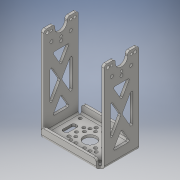
# Autodesk Inventor part: PahaAtas
Saved by Autodesk Inventor 2016 (Build 200138000, 138)
## iProperties
Created: 2017-02-10
Part Number: PahaAtas
Material: Generic
Document SubType Name: Modeling
Designer: Ghana
Density: 1 g/cm^3
Appearance: Default
Author: Ghana
Autodesk Inventor part; units mm, degrees
note: some values were not read from the file. Chosen so that the rebuilt part matches the saved one: bend side of "Bend Part10"; bend side of "Bend Part11".
ref_plane "YZ Plane" through (0, 0, 0) normal (1, 0, 0) x (0, 1, 0)
ref_plane "XZ Plane" through (0, 0, 0) normal (0, 1, 0) x (-1, 0, 0)
ref_plane "XY Plane" through (0, 0, 0) normal (0, 0, 1) x (1, 0, 0)
sketch "Sketch12" plane through (0, 0, 0) normal (0, 1, 0) x (-1, 0, 0)
  line L0 (0, 0) -> (44.454, 0)
  line L1 (44.454, 0) -> (44.454, -28)
  line L2 (44.454, -28) -> (0, -28)
  line L3 (0, -28) -> (0, 0)
  line L4 (44.454, 0) -> (46.454, 0)
  line L5 (46.454, 0) -> (46.454, -28)
  line L6 (46.454, -28) -> (44.454, -28)
  line L7 (44.454, -28) -> (44.454, 0)
  line L8 (0, 0) -> (-2, 0)
  line L9 (-2, 0) -> (-2, -28)
  line L10 (-2, -28) -> (0, -28)
  line L11 (0, -28) -> (0, 0)
  line L12 (46.454, 0) -> (115.181, 0)
  line L13 (117.181, -2) -> (117.181, -7)
  line L14 (115.181, -28) -> (46.454, -28)
  line L15 (46.454, -28) -> (46.454, 0)
  line L16 (-2, -28) -> (-70.727, -28)
  line L17 (-2, 0) -> (-2, -28)
  circle A0 centre (22.227, -14) radius 5.2
  circle A1 centre (22.227, -3) radius 1.25
  circle A2 centre (30.0052, -6.2218) radius 1.25
  circle A3 centre (33.227, -14) radius 1.25
  circle A4 centre (30.0052, -21.7782) radius 1.25
  circle A5 centre (22.227, -25) radius 1.25
  circle A6 centre (14.4488, -21.7782) radius 1.25
  circle A7 centre (11.227, -14) radius 1.25
  circle A8 centre (14.4488, -6.2218) radius 1.25
  circle A9 centre (25.727, -6) radius 1.35
  circle A10 centre (14.227, -10.5) radius 1.35
  circle A11 centre (18.727, -22) radius 1.35
  circle A12 centre (30.227, -17.5) radius 1.35
  circle A13 centre (18.727, -6) radius 1.25
  circle A14 centre (14.227, -17.5) radius 1.25
  circle A15 centre (25.727, -22) radius 1.25
  circle A16 centre (30.227, -10.5) radius 1.25
  circle A17 centre (33.227, -8) radius 1.35
  circle A18 centre (16.227, -3) radius 1.35
  circle A19 centre (11.227, -20) radius 1.35
  circle A20 centre (28.227, -25) radius 1.35
  circle A21 centre (11.227, -8) radius 1.25
  circle A22 centre (16.227, -25) radius 1.25
  circle A23 centre (33.227, -20) radius 1.25
  circle A24 centre (28.227, -3) radius 1.25
  circle A25 centre (3.227, -25) radius 1.25
  circle A26 centre (41.227, -25) radius 1.25
  circle A27 centre (3.227, -3) radius 1.25
  circle A28 centre (41.227, -3) radius 1.25
  line L18 (37.727, -9) -> (39.227, -9)
  arc A29 (40.727, -10.5) -> (39.227, -9) centre (39.227, -10.5) ccw
  line L19 (40.727, -10.5) -> (40.727, -17.5)
  arc A30 (39.227, -19) -> (40.727, -17.5) centre (39.227, -17.5) ccw
  line L20 (39.227, -19) -> (37.727, -19)
  arc A31 (36.227, -17.5) -> (37.727, -19) centre (37.727, -17.5) ccw
  line L21 (36.227, -17.5) -> (36.227, -10.5)
  arc A32 (37.727, -9) -> (36.227, -10.5) centre (37.727, -10.5) ccw
  line L22 (8.227, -10.5) -> (8.227, -17.5)
  arc A33 (6.727, -19) -> (8.227, -17.5) centre (6.727, -17.5) ccw
  line L23 (6.727, -19) -> (5.227, -19)
  arc A34 (3.727, -17.5) -> (5.227, -19) centre (5.227, -17.5) ccw
  line L24 (3.727, -17.5) -> (3.727, -10.5)
  arc A35 (5.227, -9) -> (3.727, -10.5) centre (5.227, -10.5) ccw
  line L25 (5.227, -9) -> (6.727, -9)
  arc A36 (8.227, -10.5) -> (6.727, -9) centre (6.727, -10.5) ccw
  line L26 (44.454, -28) -> (0, -28)
  line L27 (0, -28) -> (0, -30)
  line L28 (0, -30) -> (44.454, -30)
  line L29 (44.454, -30) -> (44.454, -28)
  line L30 (44.454, 0) -> (0, 0)
  line L31 (0, 0) -> (0, 2)
  line L32 (0, 2) -> (44.454, 2)
  line L33 (44.454, 2) -> (44.454, 0)
  line L34 (44.454, -30) -> (0, -30)
  line L35 (0, -30) -> (0, -33)
  line L36 (2, -35) -> (42.454, -35)
  line L37 (44.454, -33) -> (44.454, -30)
  line L38 (44.454, 2) -> (0, 2)
  line L39 (0, 2) -> (0, 5)
  line L40 (2, 7) -> (42.454, 7)
  line L41 (44.454, 5) -> (44.454, 2)
  arc A37 (42.454, -35) -> (44.454, -33) centre (42.454, -33) ccw
  arc A38 (0, -33) -> (2, -35) centre (2, -33) ccw
  arc A39 (44.454, 5) -> (42.454, 7) centre (42.454, 5) ccw
  arc A40 (2, 7) -> (0, 5) centre (2, 5) ccw
  line L42 (114.181, -19) -> (115.181, -19)
  line L43 (114.181, -9) -> (115.181, -9)
  arc A41 (114.181, -9) -> (114.181, -19) centre (114.181, -14) ccw
  line L44 (117.181, -21) -> (117.181, -26)
  circle A42 centre (114.181, -25) radius 1.25
  circle A43 centre (114.181, -22) radius 1
  circle A44 centre (106.4028, -21.7782) radius 1.25
  circle A45 centre (103.181, -14) radius 1.25
  circle A46 centre (106.4028, -6.2218) radius 1.25
  circle A47 centre (114.181, -3) radius 1.25
  circle A48 centre (106.181, -14) radius 1
  circle A49 centre (114.181, -6) radius 1
  line L45 (53.454, -8.7321) -> (53.454, -19.2679)
  line L46 (54.954, -20.134) -> (64.0784, -14.866)
  line L47 (64.0784, -13.134) -> (54.954, -7.866)
  line L48 (98.181, -19.2679) -> (98.181, -8.7321)
  line L49 (96.681, -20.134) -> (87.5566, -14.866)
  line L50 (87.5566, -13.134) -> (96.681, -7.866)
  line L51 (86.9131, -23) -> (64.7219, -23)
  line L52 (64.2219, -21.134) -> (74.8175, -15.0166)
  line L53 (76.8175, -15.0166) -> (87.4131, -21.134)
  line L54 (76.8175, -12.9834) -> (87.4131, -6.866)
  line L55 (86.9131, -5) -> (64.7219, -5)
  line L56 (64.2219, -6.866) -> (74.8175, -12.9834)
  arc A50 (74.8175, -12.9834) -> (76.8175, -12.9834) centre (75.8175, -11.2513) ccw
  arc A51 (76.8175, -15.0166) -> (74.8175, -15.0166) centre (75.8175, -16.7487) ccw
  arc A52 (96.681, -20.134) -> (98.181, -19.2679) centre (97.181, -19.2679) ccw
  arc A53 (98.181, -8.7321) -> (96.681, -7.866) centre (97.181, -8.7321) ccw
  arc A54 (87.5566, -13.134) -> (87.5566, -14.866) centre (88.0566, -14) ccw
  arc A55 (86.9131, -23) -> (87.4131, -21.134) centre (86.9131, -22) ccw
  arc A56 (64.2219, -21.134) -> (64.7219, -23) centre (64.7219, -22) ccw
  arc A57 (87.4131, -6.866) -> (86.9131, -5) centre (86.9131, -6) ccw
  arc A58 (64.7219, -5) -> (64.2219, -6.866) centre (64.7219, -6) ccw
  arc A59 (64.0784, -14.866) -> (64.0784, -13.134) centre (63.5784, -14) ccw
  arc A60 (53.454, -19.2679) -> (54.954, -20.134) centre (54.454, -19.2679) ccw
  arc A61 (54.954, -7.866) -> (53.454, -8.7321) centre (54.454, -8.7321) ccw
  line L57 (-9, -8.7321) -> (-9, -19.2679)
  line L58 (-10.5, -20.134) -> (-19.6244, -14.866)
  line L59 (-19.6244, -13.134) -> (-10.5, -7.866)
  line L60 (-53.727, -19.2679) -> (-53.727, -8.7321)
  line L61 (-52.227, -20.134) -> (-43.1026, -14.866)
  line L62 (-43.1026, -13.134) -> (-52.227, -7.866)
  line L63 (-42.4591, -23) -> (-20.2679, -23)
  line L64 (-19.7679, -21.134) -> (-30.3635, -15.0166)
  line L65 (-32.3635, -15.0166) -> (-42.9591, -21.134)
  line L66 (-32.3635, -12.9834) -> (-42.9591, -6.866)
  line L67 (-42.4591, -5) -> (-20.2679, -5)
  line L68 (-19.7679, -6.866) -> (-30.3635, -12.9834)
  arc A62 (-32.3635, -12.9834) -> (-30.3635, -12.9834) centre (-31.3635, -11.2513) ccw
  arc A63 (-30.3635, -15.0166) -> (-32.3635, -15.0166) centre (-31.3635, -16.7487) ccw
  arc A64 (-53.727, -19.2679) -> (-52.227, -20.134) centre (-52.727, -19.2679) ccw
  arc A65 (-52.227, -7.866) -> (-53.727, -8.7321) centre (-52.727, -8.7321) ccw
  arc A66 (-43.1026, -14.866) -> (-43.1026, -13.134) centre (-43.6026, -14) ccw
  arc A67 (-42.9591, -21.134) -> (-42.4591, -23) centre (-42.4591, -22) ccw
  arc A68 (-20.2679, -23) -> (-19.7679, -21.134) centre (-20.2679, -22) ccw
  arc A69 (-42.4591, -5) -> (-42.9591, -6.866) centre (-42.4591, -6) ccw
  arc A70 (-19.7679, -6.866) -> (-20.2679, -5) centre (-20.2679, -6) ccw
  arc A71 (-19.6244, -13.134) -> (-19.6244, -14.866) centre (-19.1244, -14) ccw
  arc A72 (-10.5, -20.134) -> (-9, -19.2679) centre (-10, -19.2679) ccw
  arc A73 (-9, -8.7321) -> (-10.5, -7.866) centre (-10, -8.7321) ccw
  arc A74 (115.181, -28) -> (117.181, -26) centre (115.181, -26) ccw
  arc A75 (117.181, -21) -> (115.181, -19) centre (115.181, -21) ccw
  arc A76 (115.181, -9) -> (117.181, -7) centre (115.181, -7) ccw
  arc A77 (117.181, -2) -> (115.181, 0) centre (115.181, -2) ccw
  line L69 (-72.727, -2) -> (-72.727, -7)
  line L70 (-69.727, -19) -> (-70.727, -19)
  line L71 (-69.727, -9) -> (-70.727, -9)
  arc A78 (-69.727, -19) -> (-69.727, -9) centre (-69.727, -14) ccw
  line L72 (-72.727, -21) -> (-72.727, -26)
  circle A79 centre (-69.727, -25) radius 1.25
  circle A80 centre (-69.727, -22) radius 1
  circle A81 centre (-61.9488, -21.7782) radius 1.25
  circle A82 centre (-58.727, -14) radius 1.25
  circle A83 centre (-61.9488, -6.2218) radius 1.25
  circle A84 centre (-69.727, -3) radius 1.25
  circle A85 centre (-61.727, -14) radius 1
  circle A86 centre (-69.727, -6) radius 1
  arc A87 (-72.727, -26) -> (-70.727, -28) centre (-70.727, -26) ccw
  arc A88 (-70.727, -19) -> (-72.727, -21) centre (-70.727, -21) ccw
  arc A89 (-72.727, -7) -> (-70.727, -9) centre (-70.727, -7) ccw
  arc A90 (-70.727, 0) -> (-72.727, -2) centre (-70.727, -2) ccw
  line L73 (-70.727, 0) -> (-2, 0)
  point P0 (117.181, -28)
  point P1 (117.181, 0)
  point P2 (22.227, -14)
  point P3 (0, -35)
  point P4 (0, 7)
  dimension "d88" = 2
  dimension "d89" = 2
  dimension "d91" = 70.727
  dimension "d92" = 28
  dimension "d97" = 44.454
  dimension "d98" = 2
  dimension "d99" = 44.454
  dimension "d100" = 2
  dimension "d101" = 5
  dimension "d102" = 5
  dimension "d103" = 2
  dimension "d114" = 180
  dimension "d118" = 180
  dimension "d132" = 2
  constraints: 148 end point, 92 point on circle, 91 centre point, 40 tangent, 18 parallel, 16 equal radius, 9 horizontal, 9 perpendicular, 9 point on line, 1 vertical, 14 other
  measures "d88" distance of L5.end L6.end
  measures "d89" distance of L10.end L9.end
  measures "d91" distance of point (117.181, -28) L14.end
  measures "d92" distance of point (117.181, 0) point (117.181, -28)
  measures "d97" distance of L28.end L27.end
  measures "d98" distance of L27.end L26.end
  measures "d99" distance of L31.end L32.end
  measures "d100" distance of L30.end L31.end
  measures "d101" distance of point (0, -35) L34.end
  measures "d102" distance of L38.end point (0, 7)
  measures "d103" radius of A37
  measures "d132" radius of A74
extrude "Extrusion6" add sketch "Sketch12" along normal blind 2
sketch "Sketch17" plane through (0, 2, 0) normal (0, 1, 0) x (1, 0, 0)
  arc A0 (30.3635, 15.0166) -> (32.3635, 15.0166) centre (31.3635, 16.7487) ccw projected
  line L0 (30.3635, 15.0166) -> (19.7679, 21.134) projected
  arc A1 (20.2679, 23) -> (19.7679, 21.134) centre (20.2679, 22) ccw projected
  line L1 (20.2679, 23) -> (42.4591, 23) projected
  arc A2 (42.9591, 21.134) -> (42.4591, 23) centre (42.4591, 22) ccw projected
  line L2 (42.9591, 21.134) -> (32.3635, 15.0166) projected
  arc A3 (19.7679, 6.866) -> (20.2679, 5) centre (20.2679, 6) ccw projected
  line L3 (19.7679, 6.866) -> (30.3635, 12.9834) projected
  arc A4 (32.3635, 12.9834) -> (30.3635, 12.9834) centre (31.3635, 11.2513) ccw projected
  line L4 (32.3635, 12.9834) -> (42.9591, 6.866) projected
  arc A5 (42.4591, 5) -> (42.9591, 6.866) centre (42.4591, 6) ccw projected
  line L5 (42.4591, 5) -> (20.2679, 5) projected
  arc A6 (52.227, 7.866) -> (53.727, 8.7321) centre (52.727, 8.7321) ccw projected
  line L6 (52.227, 7.866) -> (43.1026, 13.134) projected
  arc A7 (43.1026, 14.866) -> (43.1026, 13.134) centre (43.6026, 14) ccw projected
  line L7 (43.1026, 14.866) -> (52.227, 20.134) projected
  arc A8 (53.727, 19.2679) -> (52.227, 20.134) centre (52.727, 19.2679) ccw projected
  line L8 (53.727, 19.2679) -> (53.727, 8.7321) projected
  arc A9 (10.5, 20.134) -> (9, 19.2679) centre (10, 19.2679) ccw projected
  line L9 (10.5, 20.134) -> (19.6244, 14.866) projected
  arc A10 (19.6244, 13.134) -> (19.6244, 14.866) centre (19.1244, 14) ccw projected
  line L10 (19.6244, 13.134) -> (10.5, 7.866) projected
  arc A11 (9, 8.7321) -> (10.5, 7.866) centre (10, 8.7321) ccw projected
  line L11 (9, 8.7321) -> (9, 19.2679) projected
  circle A12 centre (61.9488, 6.2218) radius 1.25 projected
  circle A13 centre (69.727, 3) radius 1.25 projected
  circle A14 centre (58.727, 14) radius 1.25 projected
  circle A15 centre (69.727, 25) radius 1.25 projected
  circle A16 centre (61.9488, 21.7782) radius 1.25 projected
  circle A17 centre (69.727, 6) radius 1 projected
  circle A18 centre (61.727, 14) radius 1 projected
  circle A19 centre (69.727, 22) radius 1 projected
  arc A20 (-76.8175, 15.0166) -> (-74.8175, 15.0166) centre (-75.8175, 16.7487) ccw projected
  line L12 (-76.8175, 15.0166) -> (-87.4131, 21.134) projected
  arc A21 (-86.9131, 23) -> (-87.4131, 21.134) centre (-86.9131, 22) ccw projected
  line L13 (-86.9131, 23) -> (-64.7219, 23) projected
  arc A22 (-64.2219, 21.134) -> (-64.7219, 23) centre (-64.7219, 22) ccw projected
  line L14 (-64.2219, 21.134) -> (-74.8175, 15.0166) projected
  arc A23 (-64.7219, 5) -> (-64.2219, 6.866) centre (-64.7219, 6) ccw projected
  line L15 (-64.7219, 5) -> (-86.9131, 5) projected
  arc A24 (-87.4131, 6.866) -> (-86.9131, 5) centre (-86.9131, 6) ccw projected
  line L16 (-87.4131, 6.866) -> (-76.8175, 12.9834) projected
  arc A25 (-74.8175, 12.9834) -> (-76.8175, 12.9834) centre (-75.8175, 11.2513) ccw projected
  line L17 (-74.8175, 12.9834) -> (-64.2219, 6.866) projected
  arc A26 (-53.454, 19.2679) -> (-54.954, 20.134) centre (-54.454, 19.2679) ccw projected
  line L18 (-53.454, 19.2679) -> (-53.454, 8.7321) projected
  arc A27 (-54.954, 7.866) -> (-53.454, 8.7321) centre (-54.454, 8.7321) ccw projected
  line L19 (-54.954, 7.866) -> (-64.0784, 13.134) projected
  arc A28 (-64.0784, 14.866) -> (-64.0784, 13.134) centre (-63.5784, 14) ccw projected
  line L20 (-64.0784, 14.866) -> (-54.954, 20.134) projected
  arc A29 (-96.681, 20.134) -> (-98.181, 19.2679) centre (-97.181, 19.2679) ccw projected
  line L21 (-96.681, 20.134) -> (-87.5566, 14.866) projected
  arc A30 (-87.5566, 13.134) -> (-87.5566, 14.866) centre (-88.0566, 14) ccw projected
  line L22 (-87.5566, 13.134) -> (-96.681, 7.866) projected
  arc A31 (-98.181, 8.7321) -> (-96.681, 7.866) centre (-97.181, 8.7321) ccw projected
  line L23 (-98.181, 8.7321) -> (-98.181, 19.2679) projected
  circle A32 centre (-114.181, 3) radius 1.25 projected
  circle A33 centre (-106.4028, 6.2218) radius 1.25 projected
  circle A34 centre (-103.181, 14) radius 1.25 projected
  circle A35 centre (-106.4028, 21.7782) radius 1.25 projected
  circle A36 centre (-114.181, 25) radius 1.25 projected
  circle A37 centre (-114.181, 6) radius 1 projected
  circle A38 centre (-106.181, 14) radius 1 projected
  circle A39 centre (-114.181, 22) radius 1 projected
  circle A40 centre (-22.227, 14) radius 5.2 projected
  arc A41 (-6.727, 19) -> (-8.227, 17.5) centre (-6.727, 17.5) ccw projected
  line L24 (-6.727, 19) -> (-5.227, 19) projected
  arc A42 (-3.727, 17.5) -> (-5.227, 19) centre (-5.227, 17.5) ccw projected
  line L25 (-3.727, 17.5) -> (-3.727, 10.5) projected
  arc A43 (-5.227, 9) -> (-3.727, 10.5) centre (-5.227, 10.5) ccw projected
  line L26 (-5.227, 9) -> (-6.727, 9) projected
  arc A44 (-8.227, 10.5) -> (-6.727, 9) centre (-6.727, 10.5) ccw projected
  line L27 (-8.227, 10.5) -> (-8.227, 17.5) projected
  arc A45 (-40.727, 10.5) -> (-39.227, 9) centre (-39.227, 10.5) ccw projected
  line L28 (-40.727, 10.5) -> (-40.727, 17.5) projected
  arc A46 (-39.227, 19) -> (-40.727, 17.5) centre (-39.227, 17.5) ccw projected
  line L29 (-39.227, 19) -> (-37.727, 19) projected
  arc A47 (-36.227, 17.5) -> (-37.727, 19) centre (-37.727, 17.5) ccw projected
  line L30 (-36.227, 17.5) -> (-36.227, 10.5) projected
  arc A48 (-37.727, 9) -> (-36.227, 10.5) centre (-37.727, 10.5) ccw projected
  line L31 (-37.727, 9) -> (-39.227, 9) projected
  circle A49 centre (-28.227, 25) radius 1.35 projected
  circle A50 centre (-11.227, 20) radius 1.35 projected
  circle A51 centre (-16.227, 3) radius 1.35 projected
  circle A52 centre (-33.227, 8) radius 1.35 projected
  circle A53 centre (-30.227, 17.5) radius 1.35 projected
  circle A54 centre (-18.727, 22) radius 1.35 projected
  circle A55 centre (-14.227, 10.5) radius 1.35 projected
  circle A56 centre (-25.727, 6) radius 1.35 projected
  circle A57 centre (-41.227, 3) radius 1.25 projected
  circle A58 centre (-3.227, 3) radius 1.25 projected
  circle A59 centre (-41.227, 25) radius 1.25 projected
  circle A60 centre (-3.227, 25) radius 1.25 projected
  circle A61 centre (-28.227, 3) radius 1.25 projected
  circle A62 centre (-33.227, 20) radius 1.25 projected
  circle A63 centre (-16.227, 25) radius 1.25 projected
  circle A64 centre (-11.227, 8) radius 1.25 projected
  circle A65 centre (-30.227, 10.5) radius 1.25 projected
  circle A66 centre (-25.727, 22) radius 1.25 projected
  circle A67 centre (-14.227, 17.5) radius 1.25 projected
  circle A68 centre (-18.727, 6) radius 1.25 projected
  circle A69 centre (-14.4488, 6.2218) radius 1.25 projected
  circle A70 centre (-11.227, 14) radius 1.25 projected
  circle A71 centre (-14.4488, 21.7782) radius 1.25 projected
  circle A72 centre (-22.227, 25) radius 1.25 projected
  circle A73 centre (-30.0052, 21.7782) radius 1.25 projected
  circle A74 centre (-33.227, 14) radius 1.25 projected
  circle A75 centre (-30.0052, 6.2218) radius 1.25 projected
  circle A76 centre (-22.227, 3) radius 1.25 projected
  line L32 (-44.454, 28) -> (-115.181, 28) projected
  arc A77 (-115.181, 28) -> (-117.181, 26) centre (-115.181, 26) ccw projected
  line L33 (-117.181, 26) -> (-117.181, 21) projected
  arc A78 (-117.181, 21) -> (-115.181, 19) centre (-115.181, 21) ccw projected
  line L34 (-115.181, 19) -> (-114.181, 19) projected
  arc A79 (-114.181, 9) -> (-114.181, 19) centre (-114.181, 14) ccw projected
  line L35 (-114.181, 9) -> (-115.181, 9) projected
  arc A80 (-115.181, 9) -> (-117.181, 7) centre (-115.181, 7) ccw projected
  line L36 (-117.181, 7) -> (-117.181, 2) projected
  arc A81 (-117.181, 2) -> (-115.181, 0) centre (-115.181, 2) ccw projected
  line L37 (-115.181, 0) -> (-44.454, 0) projected
  line L38 (-44.454, 0) -> (-44.454, -5) projected
  arc A82 (-44.454, -5) -> (-42.454, -7) centre (-42.454, -5) ccw projected
  line L39 (-42.454, -7) -> (-2, -7) projected
  arc A83 (-2, -7) -> (0, -5) centre (-2, -5) ccw projected
  line L40 (0, -5) -> (0, 0) projected
  line L41 (0, 0) -> (70.727, 0) projected
  arc A84 (70.727, 0) -> (72.727, 2) centre (70.727, 2) ccw projected
  line L42 (72.727, 2) -> (72.727, 7) projected
  arc A85 (72.727, 7) -> (70.727, 9) centre (70.727, 7) ccw projected
  line L43 (70.727, 9) -> (69.727, 9) projected
  arc A86 (69.727, 19) -> (69.727, 9) centre (69.727, 14) ccw projected
  line L44 (69.727, 19) -> (70.727, 19) projected
  arc A87 (70.727, 19) -> (72.727, 21) centre (70.727, 21) ccw projected
  line L45 (72.727, 21) -> (72.727, 26) projected
  arc A88 (72.727, 26) -> (70.727, 28) centre (70.727, 26) ccw projected
  line L46 (70.727, 28) -> (0, 28) projected
  line L47 (0, 28) -> (0, 33) projected
  arc A89 (0, 33) -> (-2, 35) centre (-2, 33) ccw projected
  line L48 (-2, 35) -> (-42.454, 35) projected
  arc A90 (-42.454, 35) -> (-44.454, 33) centre (-42.454, 33) ccw projected
  line L49 (-44.454, 33) -> (-44.454, 28) projected
  line L50 (-44.454, 28) -> (-44.454, 0)
  constraints: 2 end point, 1 vertical
bend part "Bend Part9" radius 1.2732 angle 90 line through (-44.454, 2, -28) along (0, 0, 1) centre toward (0, 1, 0) moving side (-1, 0, 0) both sides no
sketch "Sketch18" plane through (0, 2, 0) normal (0, 1, 0) x (1, 0, 0)
  line L0 (-44.454, 0) -> (-44.454, 28) projected
  line L1 (-44.454, 0) -> (-44.454, -5) projected
  arc A0 (-44.454, -5) -> (-42.454, -7) centre (-42.454, -5) ccw projected
  line L2 (-42.454, -7) -> (-2, -7) projected
  arc A1 (-2, -7) -> (0, -5) centre (-2, -5) ccw projected
  line L3 (0, -5) -> (0, 0) projected
  line L4 (0, 0) -> (70.727, 0) projected
  arc A2 (70.727, 0) -> (72.727, 2) centre (70.727, 2) ccw projected
  line L5 (72.727, 2) -> (72.727, 7) projected
  arc A3 (72.727, 7) -> (70.727, 9) centre (70.727, 7) ccw projected
  line L6 (70.727, 9) -> (69.727, 9) projected
  arc A4 (69.727, 19) -> (69.727, 9) centre (69.727, 14) ccw projected
  line L7 (69.727, 19) -> (70.727, 19) projected
  arc A5 (70.727, 19) -> (72.727, 21) centre (70.727, 21) ccw projected
  line L8 (72.727, 21) -> (72.727, 26) projected
  arc A6 (72.727, 26) -> (70.727, 28) centre (70.727, 26) ccw projected
  line L9 (70.727, 28) -> (0, 28) projected
  line L10 (0, 28) -> (0, 33) projected
  arc A7 (0, 33) -> (-2, 35) centre (-2, 33) ccw projected
  line L11 (-2, 35) -> (-42.454, 35) projected
  arc A8 (-42.454, 35) -> (-44.454, 33) centre (-42.454, 33) ccw projected
  line L12 (-44.454, 33) -> (-44.454, 28) projected
  arc A9 (30.3635, 15.0166) -> (32.3635, 15.0166) centre (31.3635, 16.7487) ccw projected
  line L13 (30.3635, 15.0166) -> (19.7679, 21.134) projected
  arc A10 (20.2679, 23) -> (19.7679, 21.134) centre (20.2679, 22) ccw projected
  line L14 (20.2679, 23) -> (42.4591, 23) projected
  arc A11 (42.9591, 21.134) -> (42.4591, 23) centre (42.4591, 22) ccw projected
  line L15 (42.9591, 21.134) -> (32.3635, 15.0166) projected
  arc A12 (19.7679, 6.866) -> (20.2679, 5) centre (20.2679, 6) ccw projected
  line L16 (19.7679, 6.866) -> (30.3635, 12.9834) projected
  arc A13 (32.3635, 12.9834) -> (30.3635, 12.9834) centre (31.3635, 11.2513) ccw projected
  line L17 (32.3635, 12.9834) -> (42.9591, 6.866) projected
  arc A14 (42.4591, 5) -> (42.9591, 6.866) centre (42.4591, 6) ccw projected
  line L18 (42.4591, 5) -> (20.2679, 5) projected
  arc A15 (52.227, 7.866) -> (53.727, 8.7321) centre (52.727, 8.7321) ccw projected
  line L19 (52.227, 7.866) -> (43.1026, 13.134) projected
  arc A16 (43.1026, 14.866) -> (43.1026, 13.134) centre (43.6026, 14) ccw projected
  line L20 (43.1026, 14.866) -> (52.227, 20.134) projected
  arc A17 (53.727, 19.2679) -> (52.227, 20.134) centre (52.727, 19.2679) ccw projected
  line L21 (53.727, 19.2679) -> (53.727, 8.7321) projected
  arc A18 (10.5, 20.134) -> (9, 19.2679) centre (10, 19.2679) ccw projected
  line L22 (10.5, 20.134) -> (19.6244, 14.866) projected
  arc A19 (19.6244, 13.134) -> (19.6244, 14.866) centre (19.1244, 14) ccw projected
  line L23 (19.6244, 13.134) -> (10.5, 7.866) projected
  arc A20 (9, 8.7321) -> (10.5, 7.866) centre (10, 8.7321) ccw projected
  line L24 (9, 8.7321) -> (9, 19.2679) projected
  circle A21 centre (61.9488, 6.2218) radius 1.25 projected
  circle A22 centre (69.727, 3) radius 1.25 projected
  circle A23 centre (58.727, 14) radius 1.25 projected
  circle A24 centre (69.727, 25) radius 1.25 projected
  circle A25 centre (61.9488, 21.7782) radius 1.25 projected
  circle A26 centre (69.727, 6) radius 1 projected
  circle A27 centre (61.727, 14) radius 1 projected
  circle A28 centre (69.727, 22) radius 1 projected
  circle A29 centre (-22.227, 14) radius 5.2 projected
  arc A30 (-6.727, 19) -> (-8.227, 17.5) centre (-6.727, 17.5) ccw projected
  line L25 (-6.727, 19) -> (-5.227, 19) projected
  arc A31 (-3.727, 17.5) -> (-5.227, 19) centre (-5.227, 17.5) ccw projected
  line L26 (-3.727, 17.5) -> (-3.727, 10.5) projected
  arc A32 (-5.227, 9) -> (-3.727, 10.5) centre (-5.227, 10.5) ccw projected
  line L27 (-5.227, 9) -> (-6.727, 9) projected
  arc A33 (-8.227, 10.5) -> (-6.727, 9) centre (-6.727, 10.5) ccw projected
  line L28 (-8.227, 10.5) -> (-8.227, 17.5) projected
  arc A34 (-40.727, 10.5) -> (-39.227, 9) centre (-39.227, 10.5) ccw projected
  line L29 (-40.727, 10.5) -> (-40.727, 17.5) projected
  arc A35 (-39.227, 19) -> (-40.727, 17.5) centre (-39.227, 17.5) ccw projected
  line L30 (-39.227, 19) -> (-37.727, 19) projected
  arc A36 (-36.227, 17.5) -> (-37.727, 19) centre (-37.727, 17.5) ccw projected
  line L31 (-36.227, 17.5) -> (-36.227, 10.5) projected
  arc A37 (-37.727, 9) -> (-36.227, 10.5) centre (-37.727, 10.5) ccw projected
  line L32 (-37.727, 9) -> (-39.227, 9) projected
  circle A38 centre (-28.227, 25) radius 1.35 projected
  circle A39 centre (-11.227, 20) radius 1.35 projected
  circle A40 centre (-16.227, 3) radius 1.35 projected
  circle A41 centre (-33.227, 8) radius 1.35 projected
  circle A42 centre (-30.227, 17.5) radius 1.35 projected
  circle A43 centre (-18.727, 22) radius 1.35 projected
  circle A44 centre (-14.227, 10.5) radius 1.35 projected
  circle A45 centre (-25.727, 6) radius 1.35 projected
  circle A46 centre (-41.227, 3) radius 1.25 projected
  circle A47 centre (-3.227, 3) radius 1.25 projected
  circle A48 centre (-41.227, 25) radius 1.25 projected
  circle A49 centre (-3.227, 25) radius 1.25 projected
  circle A50 centre (-28.227, 3) radius 1.25 projected
  circle A51 centre (-33.227, 20) radius 1.25 projected
  circle A52 centre (-16.227, 25) radius 1.25 projected
  circle A53 centre (-11.227, 8) radius 1.25 projected
  circle A54 centre (-30.227, 10.5) radius 1.25 projected
  circle A55 centre (-25.727, 22) radius 1.25 projected
  circle A56 centre (-14.227, 17.5) radius 1.25 projected
  circle A57 centre (-18.727, 6) radius 1.25 projected
  circle A58 centre (-14.4488, 6.2218) radius 1.25 projected
  circle A59 centre (-11.227, 14) radius 1.25 projected
  circle A60 centre (-14.4488, 21.7782) radius 1.25 projected
  circle A61 centre (-22.227, 25) radius 1.25 projected
  circle A62 centre (-30.0052, 21.7782) radius 1.25 projected
  circle A63 centre (-33.227, 14) radius 1.25 projected
  circle A64 centre (-30.0052, 6.2218) radius 1.25 projected
  circle A65 centre (-22.227, 3) radius 1.25 projected
  line L33 (0, 28) -> (0, 0)
  constraints: 2 end point, 1 vertical
bend part "Bend Part10" radius 1.2732 angle 90 line through (0, 2, -28) along (0, 0, 1) centre toward (0, 1, 0) moving side (1, 0, 0) both sides no
sketch "Sketch19" plane through (0, 2, 0) normal (0, 1, 0) x (1, 0, 0)
  circle A0 centre (-22.227, 3) radius 1.25 projected
  circle A1 centre (-30.0052, 6.2218) radius 1.25 projected
  circle A2 centre (-33.227, 14) radius 1.25 projected
  circle A3 centre (-30.0052, 21.7782) radius 1.25 projected
  circle A4 centre (-22.227, 25) radius 1.25 projected
  circle A5 centre (-14.4488, 21.7782) radius 1.25 projected
  circle A6 centre (-11.227, 14) radius 1.25 projected
  circle A7 centre (-14.4488, 6.2218) radius 1.25 projected
  circle A8 centre (-18.727, 6) radius 1.25 projected
  circle A9 centre (-14.227, 17.5) radius 1.25 projected
  circle A10 centre (-25.727, 22) radius 1.25 projected
  circle A11 centre (-30.227, 10.5) radius 1.25 projected
  circle A12 centre (-11.227, 8) radius 1.25 projected
  circle A13 centre (-16.227, 25) radius 1.25 projected
  circle A14 centre (-33.227, 20) radius 1.25 projected
  circle A15 centre (-28.227, 3) radius 1.25 projected
  circle A16 centre (-3.227, 25) radius 1.25 projected
  circle A17 centre (-41.227, 25) radius 1.25 projected
  circle A18 centre (-3.227, 3) radius 1.25 projected
  circle A19 centre (-41.227, 3) radius 1.25 projected
  circle A20 centre (-25.727, 6) radius 1.35 projected
  circle A21 centre (-14.227, 10.5) radius 1.35 projected
  circle A22 centre (-18.727, 22) radius 1.35 projected
  circle A23 centre (-30.227, 17.5) radius 1.35 projected
  circle A24 centre (-33.227, 8) radius 1.35 projected
  circle A25 centre (-16.227, 3) radius 1.35 projected
  circle A26 centre (-11.227, 20) radius 1.35 projected
  circle A27 centre (-28.227, 25) radius 1.35 projected
  arc A28 (-40.727, 10.5) -> (-39.227, 9) centre (-39.227, 10.5) ccw projected
  line L0 (-40.727, 10.5) -> (-40.727, 17.5) projected
  arc A29 (-39.227, 19) -> (-40.727, 17.5) centre (-39.227, 17.5) ccw projected
  line L1 (-39.227, 19) -> (-37.727, 19) projected
  arc A30 (-36.227, 17.5) -> (-37.727, 19) centre (-37.727, 17.5) ccw projected
  line L2 (-36.227, 17.5) -> (-36.227, 10.5) projected
  arc A31 (-37.727, 9) -> (-36.227, 10.5) centre (-37.727, 10.5) ccw projected
  line L3 (-37.727, 9) -> (-39.227, 9) projected
  arc A32 (-6.727, 19) -> (-8.227, 17.5) centre (-6.727, 17.5) ccw projected
  line L4 (-6.727, 19) -> (-5.227, 19) projected
  arc A33 (-3.727, 17.5) -> (-5.227, 19) centre (-5.227, 17.5) ccw projected
  line L5 (-3.727, 17.5) -> (-3.727, 10.5) projected
  arc A34 (-5.227, 9) -> (-3.727, 10.5) centre (-5.227, 10.5) ccw projected
  line L6 (-5.227, 9) -> (-6.727, 9) projected
  arc A35 (-8.227, 10.5) -> (-6.727, 9) centre (-6.727, 10.5) ccw projected
  line L7 (-8.227, 10.5) -> (-8.227, 17.5) projected
  circle A36 centre (-22.227, 14) radius 5.2 projected
  line L8 (0, 28) -> (0, 0) projected
  line L9 (0, 28) -> (0, 33) projected
  arc A37 (0, 33) -> (-2, 35) centre (-2, 33) ccw projected
  line L10 (-2, 35) -> (-42.454, 35) projected
  arc A38 (-42.454, 35) -> (-44.454, 33) centre (-42.454, 33) ccw projected
  line L11 (-44.454, 33) -> (-44.454, 28) projected
  line L12 (-44.454, 0) -> (-44.454, 28) projected
  line L13 (-44.454, 0) -> (-44.454, -5) projected
  arc A39 (-44.454, -5) -> (-42.454, -7) centre (-42.454, -5) ccw projected
  line L14 (-42.454, -7) -> (-2, -7) projected
  arc A40 (-2, -7) -> (0, -5) centre (-2, -5) ccw projected
  line L15 (0, -5) -> (0, 0) projected
  line L16 (-44.454, 28) -> (0, 28)
  constraints: 2 end point, 1 horizontal
bend part "Bend Part11" radius 1.2732 angle 90 line through (-44.454, 2, -28) along (1, 0, 0) centre toward (0, 1, 0) moving side (0, 0, -1) both sides no
sketch "Sketch20" plane through (0, 2, 0) normal (0, 1, 0) x (1, 0, 0)
  line L0 (-44.454, 28) -> (0, 28) projected
  line L1 (-44.454, 0) -> (-44.454, 28) projected
  line L2 (-44.454, 0) -> (-44.454, -5) projected
  arc A0 (-44.454, -5) -> (-42.454, -7) centre (-42.454, -5) ccw projected
  line L3 (-42.454, -7) -> (-2, -7) projected
  arc A1 (-2, -7) -> (0, -5) centre (-2, -5) ccw projected
  line L4 (0, -5) -> (0, 0) projected
  line L5 (0, 28) -> (0, 0) projected
  circle A2 centre (-22.227, 14) radius 5.2 projected
  arc A3 (-6.727, 19) -> (-8.227, 17.5) centre (-6.727, 17.5) ccw projected
  line L6 (-6.727, 19) -> (-5.227, 19) projected
  arc A4 (-3.727, 17.5) -> (-5.227, 19) centre (-5.227, 17.5) ccw projected
  line L7 (-3.727, 17.5) -> (-3.727, 10.5) projected
  arc A5 (-5.227, 9) -> (-3.727, 10.5) centre (-5.227, 10.5) ccw projected
  line L8 (-5.227, 9) -> (-6.727, 9) projected
  arc A6 (-8.227, 10.5) -> (-6.727, 9) centre (-6.727, 10.5) ccw projected
  line L9 (-8.227, 10.5) -> (-8.227, 17.5) projected
  arc A7 (-40.727, 10.5) -> (-39.227, 9) centre (-39.227, 10.5) ccw projected
  line L10 (-40.727, 10.5) -> (-40.727, 17.5) projected
  arc A8 (-39.227, 19) -> (-40.727, 17.5) centre (-39.227, 17.5) ccw projected
  line L11 (-39.227, 19) -> (-37.727, 19) projected
  arc A9 (-36.227, 17.5) -> (-37.727, 19) centre (-37.727, 17.5) ccw projected
  line L12 (-36.227, 17.5) -> (-36.227, 10.5) projected
  arc A10 (-37.727, 9) -> (-36.227, 10.5) centre (-37.727, 10.5) ccw projected
  line L13 (-37.727, 9) -> (-39.227, 9) projected
  circle A11 centre (-28.227, 25) radius 1.35 projected
  circle A12 centre (-11.227, 20) radius 1.35 projected
  circle A13 centre (-16.227, 3) radius 1.35 projected
  circle A14 centre (-33.227, 8) radius 1.35 projected
  circle A15 centre (-30.227, 17.5) radius 1.35 projected
  circle A16 centre (-18.727, 22) radius 1.35 projected
  circle A17 centre (-14.227, 10.5) radius 1.35 projected
  circle A18 centre (-25.727, 6) radius 1.35 projected
  circle A19 centre (-41.227, 3) radius 1.25 projected
  circle A20 centre (-3.227, 3) radius 1.25 projected
  circle A21 centre (-41.227, 25) radius 1.25 projected
  circle A22 centre (-3.227, 25) radius 1.25 projected
  circle A23 centre (-28.227, 3) radius 1.25 projected
  circle A24 centre (-33.227, 20) radius 1.25 projected
  circle A25 centre (-16.227, 25) radius 1.25 projected
  circle A26 centre (-11.227, 8) radius 1.25 projected
  circle A27 centre (-30.227, 10.5) radius 1.25 projected
  circle A28 centre (-25.727, 22) radius 1.25 projected
  circle A29 centre (-14.227, 17.5) radius 1.25 projected
  circle A30 centre (-18.727, 6) radius 1.25 projected
  circle A31 centre (-14.4488, 6.2218) radius 1.25 projected
  circle A32 centre (-11.227, 14) radius 1.25 projected
  circle A33 centre (-14.4488, 21.7782) radius 1.25 projected
  circle A34 centre (-22.227, 25) radius 1.25 projected
  circle A35 centre (-30.0052, 21.7782) radius 1.25 projected
  circle A36 centre (-33.227, 14) radius 1.25 projected
  circle A37 centre (-30.0052, 6.2218) radius 1.25 projected
  circle A38 centre (-22.227, 3) radius 1.25 projected
  line L14 (-44.454, 0) -> (0, 0)
  constraints: 2 end point, 1 horizontal
bend part "Bend Part12" radius 1.2732 angle 90 line through (-44.454, 2, 0) along (1, 0, 0) centre toward (0, 1, 0) moving side (0, 0, 1) both sides no
body "Solid4"
